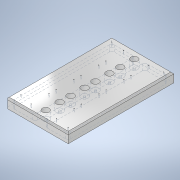
# Autodesk Inventor part: Assembly Plate
Saved by Autodesk Inventor 2022 (Build 260153000, 153)
## iProperties
Created: 2022-03-23
Part Number: Assembly Plate
Material: Generic
Document SubType Name: Modeling
Designer: Caleb
Density: 1 g/cm^3
Appearance: Aluminum - Dark
Author: Caleb
Autodesk Inventor part; units mm, degrees
ref_plane "YZ Plane" through (0, 0, 0) normal (1, 0, 0) x (0, 1, 0)
ref_plane "XZ Plane" through (0, 0, 0) normal (0, 1, 0) x (-1, 0, 0)
ref_plane "XY Plane" through (0, 0, 0) normal (0, 0, 1) x (1, 0, 0)
sketch "Sketch1" plane through (0, 0, 0) normal (0, 1, 0) x (-1, 0, 0)
  line L0 (-63.5, -107.95) -> (63.5, -107.95)
  line L1 (63.5, -107.95) -> (63.5, 107.95)
  line L2 (63.5, 107.95) -> (-63.5, 107.95)
  line L3 (-63.5, 107.95) -> (-63.5, -107.95)
  line L4 (-63.5, -107.95) -> (63.5, 107.95) construction
  line L5 (63.5, -107.95) -> (-63.5, 107.95) construction
  point P0 (0, 0)
  dimension "d0" = 127
  dimension "d1" = 215.9
  constraints: 12 end point, 2 midpoint, 2 parallel, 1 horizontal, 1 perpendicular
  measures "d0" distance of L2.end L1.end
  measures "d1" distance of L1.end L0.end
extrude "Extrusion1" add sketch "Sketch1" along normal blind 19.05
sketch "Sketch4" plane through (0, 19.05, 0) normal (0, 1, 0) x (1, 0, 0)
  line L0 (-63.5, -107.95) -> (63.5, -107.95) projected
  line L1 (-63.5, 107.95) -> (-63.5, -107.95) projected
  point P0 (0, 0)
  point P1 (0, -90.5002)
  point P2 (0, -61.8871)
  point P3 (0, -11.0871)
  point P4 (0, -39.7002)
  point P5 (0, 39.7129)
  point P6 (0, 11.0998)
  point P7 (0, 90.5129)
  point P8 (0, 61.8998)
  dimension "d14" = 17.4498
  dimension "d15" = 46.0629
  dimension "d18" = 50.8
  constraints: 1 vertical, 6 other
  measures "d14" distance from line of L0 point (0, -90.5)
  measures "d15" distance from line of L0 point (0, -61.887)
  measures "d18" distance of point (0, -61.887) point (0, -11.087)
hole "Hole2" at (0, 19.05, 90.5002) at (0, 19.05, 61.8871) at (0, 19.05, 11.0871) at (0, 19.05, 39.7002) at (0, 19.05, -39.7129) at (0, 19.05, -11.0998) at (0, 19.05, -90.5129) at (0, 19.05, -61.8998) direction (0, -1, 0) diameter 3.9624 end through all counterbore diameter 13.97 counterbore depth 15.24 thread size "10-32 UNF" class "2B" standard "ANSI Unified Screw Threads"
sketch "Sketch5" plane through (0, 19.05, 0) normal (0, 1, 0) x (1, 0, 0)
  line L0 (-63.5, -107.95) -> (63.5, -107.95) projected
  line L1 (63.5, 107.95) -> (-63.5, 107.95) projected
  line L2 (-63.5, 107.95) -> (-63.5, -107.95) projected
  line L3 (63.5, -107.95) -> (63.5, 107.95) projected
  point P0 (0, 0)
  point P1 (-53.15, -87.9)
  point P2 (-53.15, 97.6)
  point P3 (53.15, 97.6)
  point P4 (53.15, -97.6)
  dimension "d31" = 20.05
  dimension "d32" = 10.35
  dimension "d33" = 10.35
  dimension "d34" = 10.35
  dimension "d35" = 10.35
  dimension "d36" = 10.35
  dimension "d37" = 10.35
  dimension "d38" = 10.35
  measures "d31" distance from line of L0 point (-53.15, -87.9)
  measures "d32" distance from line of L0 point (53.15, -97.6)
  measures "d33" distance from line of L1 point (53.15, 97.6)
  measures "d34" distance from line of L1 point (-53.15, 97.6)
  measures "d35" distance from line of L2 point (-53.15, 97.6)
  measures "d36" distance from line of L3 point (53.15, 97.6)
  measures "d37" distance from line of L3 point (53.15, -97.6)
  measures "d38" distance from line of L2 point (-53.15, -87.9)
hole "Hole3" at (-53.15, 19.05, 87.9) at (-53.15, 19.05, -97.6) at (53.15, 19.05, -97.6) at (53.15, 19.05, 97.6) direction (0, -1, 0) diameter 1.0211 end through all thread size "00-96 NS" class "2B" standard "ANSI Unified Screw Threads"
sketch "Sketch6" plane through (0, 19.05, 0) normal (0, 1, 0) x (1, 0, 0)
  line L0 (-63.5, -107.95) -> (63.5, -107.95) projected
  line L1 (-63.5, 107.95) -> (-63.5, -107.95) projected
  point P0 (0, 0)
  point P1 (-25.75, -94.25)
  point P2 (-25.75, -58.15)
  point P3 (25.75, -58.15)
  point P4 (25.75, -94.25)
  point P5 (25.75, -43.45)
  point P6 (25.75, -7.35)
  point P7 (-25.75, -7.35)
  point P8 (-25.75, -43.45)
  point P9 (25.75, 7.35)
  point P10 (25.75, 43.45)
  point P11 (-25.75, 43.45)
  point P12 (-25.75, 7.35)
  point P13 (25.75, 58.15)
  point P14 (25.75, 94.25)
  point P15 (-25.75, 94.25)
  point P16 (-25.75, 58.15)
  dimension "d46" = 36.1
  dimension "d47" = 51.5
  dimension "d48" = 13.7
  dimension "d49" = 37.75
  dimension "d52" = 50.8
  constraints: 2 horizontal alignment, 2 vertical alignment, 1 vertical, 12 other
  measures "d46" distance of point (-25.75, -58.15) point (-25.75, -94.25)
  measures "d47" distance of point (25.75, -94.25) point (-25.75, -94.25)
  measures "d48" distance from line of L0 point (-25.75, -94.25)
  measures "d49" distance from line of L1 point (-25.75, -94.25)
  measures "d52" distance of point (25.75, -94.25) point (25.75, -43.45)
hole "Hole4" at (-25.75, 19.05, 94.25) at (-25.75, 19.05, 58.15) at (25.75, 19.05, 58.15) at (25.75, 19.05, 94.25) at (25.75, 19.05, 43.45) at (25.75, 19.05, 7.35) at (-25.75, 19.05, 7.35) at (-25.75, 19.05, 43.45) at (25.75, 19.05, -7.35) at (25.75, 19.05, -43.45) at (-25.75, 19.05, -43.45) at (-25.75, 19.05, -7.35) at (25.75, 19.05, -58.15) at (25.75, 19.05, -94.25) at (-25.75, 19.05, -94.25) at (-25.75, 19.05, -58.15) direction (0, -1, 0) diameter 1.1811 end through all thread size "0-80 UNF" class "2B" standard "ANSI Unified Screw Threads"
chamfer "Chamfer1" distance 3.175 angle 45 2 edges at (0, 19.05, 107.95) (63.5, 19.05, 0)
chamfer "Chamfer2" distance 3.175 angle 45 3 edges at (-1.5875, 19.05, -107.95) (-63.5, 19.05, -1.5875) (-63.5, 7.9375, 107.95)
sketch "Sketch7" plane through (0, 0, 0) normal (0, -1, 0) x (1, 0, 0)
  line L0 (15, 101.6) -> (52.15, 101.6)
  line L1 (57.15, 96.6) -> (57.15, -96.6)
  line L2 (52.15, -101.6) -> (15, -101.6)
  line L3 (10, -96.6) -> (10, 96.6)
  line L4 (63.5, 107.95) -> (63.5, -107.95) projected
  line L5 (-60.325, 107.95) -> (63.5, 107.95) projected
  line L6 (63.5, -107.95) -> (-63.5, -107.95) projected
  circle A0 centre (0, 90.5002) radius 1.9812 projected
  arc A1 (15, 101.6) -> (10, 96.6) centre (15, 96.6) ccw
  arc A2 (57.15, 96.6) -> (52.15, 101.6) centre (52.15, 96.6) ccw
  arc A3 (52.15, -101.6) -> (57.15, -96.6) centre (52.15, -96.6) ccw
  arc A4 (10, -96.6) -> (15, -101.6) centre (15, -96.6) ccw
  line L7 (-60.325, 107.95) -> (63.5, 107.95) construction
  line L8 (0, 107.95) -> (0, -107.95) construction
  line L9 (-15, 101.6) -> (-52.15, 101.6)
  line L10 (-57.15, 96.6) -> (-57.15, -96.6)
  line L11 (-52.15, -101.6) -> (-15, -101.6)
  line L12 (-10, -96.6) -> (-10, 96.6)
  arc A5 (-10, 96.6) -> (-15, 101.6) centre (-15, 96.6) ccw
  arc A6 (-52.15, 101.6) -> (-57.15, 96.6) centre (-52.15, 96.6) ccw
  arc A7 (-57.15, -96.6) -> (-52.15, -101.6) centre (-52.15, -96.6) ccw
  arc A8 (-15, -101.6) -> (-10, -96.6) centre (-15, -96.6) ccw
  point P0 (0, 0)
  dimension "d70" = 6.35
  dimension "d71" = 6.35
  dimension "d72" = 6.35
  dimension "d73" = 10
  dimension "d74" = 5
  constraints: 18 end point, 16 point on circle, 12 symmetric about line, 8 centre point, 8 tangent, 3 equal radius, 2 parallel, 1 horizontal, 1 midpoint, 1 perpendicular, 1 point on line, 4 other
  measures "d70" distance between parallel lines of L4 L1
  measures "d71" distance between parallel lines of L5 L0
  measures "d72" distance between parallel lines of L6 L2
  measures "d73" distance from line of L3 A0.centre
  measures "d74" radius of A1
extrude "Extrusion3" cut sketch "Sketch7" against normal blind 12.7 contours L0 A2 L1 A3 L2 A4 L3 A1 | A5 L12 A8 L11 A7 L10 A6 L9
equation "\"d71\" = d70"
equation "\"d72\" = d70"
body "Solid1"
